Motor_v3 (Autodesk Fusion 360 design; units mm, degrees)
Autodesk Fusion 360 part; units mm, degrees
sketch "Sketch1" plane through (0, 0, 0) normal (0, 0, 1) x (1, 0, 0)
  circle A0 centre (0, 0) radius 34
  dimension "MotorDia" = 68
  constraint coincident A0.centre origin
  measures "MotorDia" diameter of A0
extrude "Extrude1" add sketch "Sketch1" along normal blind 33.8
chamfer "Chamfer1" distance 4 distance2 9 1 edges at (-31.6991, -12.2949, 0) measured on face at (33.9577, -1.6948, 22.5333)
chamfer "Chamfer2" distance 20 distance2 9 1 edges at (-31.6991, -12.2949, 33.8) measured on face at (10.8298, 6.4941, 33.8)
